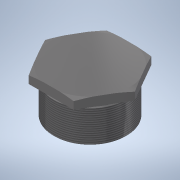
# Autodesk Inventor part: Korek sześciokątny BSP 3'' L=54
Saved by Autodesk Inventor 2020 (Build 240168000, 168)
## iProperties
RuleStatus: InUse
Created: 2022-03-21
Part Number: Korek sześciokątny BSP 3'' L=54
Material: 304
Description: Korek sześciokątny BSP 3'' L=54
Document SubType Name: Modelowanie
Designer: Radosław
Density: 8 g/cm^3
Sheet Metal Rule: 1,5
Sheet Metal Width: 0,000 mm
Sheet Metal Length: 0,000 mm
Sheet Metal Area: 0,000 mm^2
Appearance: Częściowo polerowany(1)
Author: Radosław
Autodesk Inventor part; units mm, degrees
ref_plane "YZ Plane" through (0, 0, 0) normal (1, 0, 0) x (0, 1, 0)
ref_plane "XZ Plane" through (0, 0, 0) normal (0, 1, 0) x (-1, 0, 0)
ref_plane "XY Plane" through (0, 0, 0) normal (0, 0, 1) x (1, 0, 0)
sketch "Szkic7" plane through (0, 0, 0) normal (0, 0, 1) x (1, 0, 0)
  circle A0 centre (0, 0) radius 43.942
  dimension "d35" = 87.884
  constraints: 1 centre point, 1 coincident
  measures "d35" diameter of A0
extrude "Wyciągnięcie proste2" add sketch "Szkic7" along normal mid plane 39.825
chamfer "Faza2" distance 1 angle 45 1 edges at (-43.942, 0, 19.9125)
sketch "Szkic9" plane through (0, 0, 19.9125) normal (0, 0, 1) x (1, 0, 0)
  circle A0 centre (0, 0) radius 42.942 projected
extrude "Wyciągnięcie proste3" add sketch "Szkic9" along normal blind 3.375
sketch "Szkic10" plane through (0, 0, 23.2875) normal (0, 0, 1) x (1, 0, 0)
  line L0 (-27.1355, 47) -> (27.1355, 47)
  line L1 (27.1355, 47) -> (54.2709, 0)
  line L2 (54.2709, 0) -> (27.1355, -47)
  line L3 (27.1355, -47) -> (-27.1355, -47)
  line L4 (-27.1355, -47) -> (-54.2709, 0)
  line L5 (-54.2709, 0) -> (-27.1355, 47)
  line L6 (0, 61.5188) -> (0, -61.5188) construction
  line L7 (-61.5188, 0) -> (61.5188, 0) construction
  point P0 (0, 0)
  point P1 (0, 0)
  point P2 (0, 47)
  dimension "d44" = 94
  constraints: 12 end point, 2 point on line, 1 coincident, 1 midpoint, 13 other
  measures "d44" distance between parallel lines of L4 L1
extrude "Wyciągnięcie proste4" add sketch "Szkic10" along normal blind 10.8
sketch "Szkic12" plane through (0, 0, 0) normal (0, 1, 0) x (-1, 0, 0)
  line L0 (0, -2.1463) -> (0, 12.8775) construction
  line L1 (-27.1355, 23.2875) -> (-27.1355, 34.0875) construction
  line L2 (-54.2709, 34.0875) -> (-27.1355, 34.0875) construction
  line L3 (-54.2709, 23.2875) -> (-54.2709, 34.0875) projected
  line L4 (-54.2709, 32.4084) -> (-48.0043, 34.0875)
  line L5 (-54.2709, 34.0875) -> (-27.1355, 34.0875) projected
  line L6 (-54.2709, 23.2875) -> (-27.1355, 23.2875) projected
  point P0 (0, 0)
  dimension "d50" = 15
  dimension "d51" = 6.2667
  constraints: 2 end point, 2 point on line
  measures "d50" angle of L2 L4
  measures "d51" distance from line of L3 L4.end
revolve "Obrót2" cut sketch "Szkic12" angle 360 about axis through (0, 0, -10) along (0, 0, 1)
thread "Gwint3" size "G87.884x2.309" designation "G 3" class "A" standard "ISO Pipe Threads" full length
chamfer "Faza3" distance 1 angle 45 1 edges at (-43.942, 0, -19.9125)
equation "\"d35\" = OD"
equation "\"d36\" = 0.7375 * L"
equation "\"d42\" = 0.0625 * L"
equation "\"d44\" = SW"
equation "\"d45\" = 0.2 * L"
equation "\"d51\" = 0.0666667 * SW"
equation "\"SzerokośćGięciaPodcięcia\" = Grubość"
equation "\"RozmiarPodcięciaNarożnika\" = 4 * Grubość"
equation "\"PromieńPrzejścia\" = PromieńGięcia"
equation "\"Rozmiar_promienia_Jacobiego\" = PromieńGięcia"
equation "\"Wielk_odstępu\" = Grubość"
equation "\"d2\" = PromieńGięcia"
equation "\"d23\" = PromieńGięcia"
equation "\"OD\" = 87.884"
equation "\"SW\" = 94"
equation "\"L\" = 54"
equation "\"Grubość\" = 1.5"
equation "\"PromieńGięcia\" = 3"
